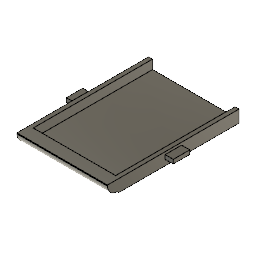
puhelimen paikka EI tappeja v1 (Autodesk Fusion 360 design; units mm, degrees)
Autodesk Fusion 360 part; units mm, degrees
sketch "Sketch1" plane through (0, 0, 0) normal (0, 0, 1) x (1, 0, 0)
  line L0 (-50, 80) -> (60, 80)
  line L1 (60, 80) -> (60, -80)
  line L2 (60, -80) -> (-50, -80)
  line L3 (-50, -80) -> (-50, 80)
  dimension "d1" = 110
  dimension "d2" = 160
  constraint horizontal L0
  constraint vertical L1
  constraint horizontal L2
  constraint vertical L3
  measures "d1" distance of L0.start L0.end
  measures "d2" distance of L0.start L2.end
extrude "Extrude1" add sketch "Sketch1" along normal blind 12
sketch "Sketch2" plane through (0, 0, 12) normal (0, 0, 1) x (-1, 0, 0)
  line L0 (50, 80) -> (-60, 80)
  line L1 (-60, 80) -> (-60, -80)
  line L2 (-60, -80) -> (50, -80)
  line L3 (50, -80) -> (50, 80)
  line L4 (45, -80) -> (-55, -80)
  line L5 (-55, -80) -> (-55, 70)
  line L6 (-55, 70) -> (45, 70)
  line L7 (45, 70) -> (45, -80)
  constraint horizontal L4
  constraint vertical L5
  constraint horizontal L6
  constraint vertical L7
  constraint coincident L2 L4.start
extrude "Extrude2" cut sketch "Sketch2" against normal blind 10 contours L2 L4 L5 L6 L7
sketch "Sketch3" plane through (0, -70, 0) normal (0, 1, 0) x (-1, 0, 0)
  line L0 (45, 12) -> (-55, 12)
  line L1 (-55, 12) -> (-55, 2)
  line L2 (-55, 2) -> (45, 2)
  line L3 (45, 2) -> (45, 12)
  line L4 (-55, 12) -> (45, 12)
  line L5 (45, 12) -> (45, 11)
  line L6 (45, 11) -> (-55, 11)
  line L7 (-55, 11) -> (-55, 12)
  dimension "d7" = 1
  constraint horizontal L4
  constraint vertical L5
  constraint horizontal L6
  constraint vertical L7
  constraint coincident L0.end L1.start
  measures "d7" distance of L0.end L6.end
extrude "Extrude3" add sketch "Sketch3" along normal blind 5 contours L0 L1 L3 L4 L5 L6 L7
fillet "Fillet1" radius 12 1 edges at (5, -80, 0)
sketch "Sketch4" plane through (60, 0, 0) normal (1, 0, 0) x (0, 1, 0)
  arc A0 (-80, 12) -> (-68, 0) centre (-68, 12) ccw
  line L0 (-68, 0) -> (80, 0)
  line L1 (80, 0) -> (80, 12)
  line L2 (80, 12) -> (-80, 12)
  line L3 (-10, 10) -> (10, 10)
  line L4 (10, 10) -> (10, 5)
  line L5 (10, 5) -> (-10, 5)
  line L6 (-10, 5) -> (-10, 10)
  dimension "d12" = 20
  constraint horizontal L3
  constraint vertical L4
  constraint horizontal L5
  constraint vertical L6
  measures "d12" distance of L3.start L3.end
extrude "Extrude4" add sketch "Sketch4" along normal blind 10 contours L3 L4 L5 L6
sketch "Sketch5" plane through (-50, 0, 0) normal (-1, 0, 0) x (0, -1, 0)
  arc A0 (68, 0) -> (80, 12) centre (68, 12) ccw
  line L0 (80, 12) -> (-80, 12)
  line L1 (-80, 12) -> (-80, 0)
  line L2 (-80, 0) -> (68, 0)
  line L3 (-10, 10) -> (10, 10)
  line L4 (10, 10) -> (10, 5)
  line L5 (10, 5) -> (-10, 5)
  line L6 (-10, 5) -> (-10, 10)
  dimension "d15" = 20
  constraint horizontal L3
  constraint vertical L4
  constraint horizontal L5
  constraint vertical L6
  measures "d15" distance of L3.start L3.end
extrude "Extrude5" add sketch "Sketch5" along normal blind 10 contours L3 L4 L5 L6
extrude "Extrude6" add 1 faces at (21.6667, -75, 12) along direction (0, 0, 1) blind 1
extrude "Extrude7" add 1 faces at (-13.3333, -18.6683, 0) along direction (0, 0, -1) blind 2
fillet "Fillet2" radius 3 1 edges at (5, -68, -2)
